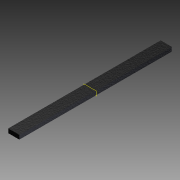
# Autodesk Inventor part: Foam_001
Saved by Autodesk Inventor 2015 (Build 190159000, 159)
## iProperties
Created: 2014-03-13
Part Number: Foam_001
Document SubType Name: Modeling
Designer: Oscar
Density: 1 g/cm^3
Material: Generic
Appearance: Black Cast
Author: Oscar
Autodesk Inventor part; units mm, degrees
ref_plane "YZ Plane" through (0, 0, 0) normal (1, 0, 0) x (0, 1, 0)
ref_plane "XY Plane" through (0, 0, 0) normal (0, 0, 1) x (1, 0, 0)
sketch "Boceto1" plane through (0, 0, 0) normal (0, 0, 1) x (1, 0, 0)
  line L0 (4.75, 65) -> (-4.75, 65)
  line L1 (-4.75, 65) -> (-4.75, -65)
  line L2 (-4.75, -65) -> (4.75, -65)
  line L3 (4.75, -65) -> (4.75, 65)
  point P0 (0, 0)
  point P1 (4.75, 0)
  point P2 (0, 65)
  dimension "d0" = 9.5
  dimension "d1" = 130
  constraints: 8 end point, 2 midpoint, 2 parallel, 1 horizontal, 1 horizontal alignment, 1 perpendicular, 1 vertical alignment
  measures "d0" distance of L1.end L2.end
  measures "d1" distance of L2.end L0.start
extrude "Extrusión1" add sketch "Boceto1" along normal blind 3.5
body "Solid1"
